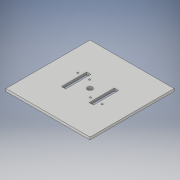
# Autodesk Inventor part: thumper-bumper-base
Saved by Autodesk Inventor 2017 (Build 210142000, 142)
## iProperties
Created: 2017-02-21
Part Number: thumper-bumper-base
Material: Generic
Document SubType Name: Modeling
Designer: John
Density: 1 g/cm^3
Appearance: Default
Author: John
Autodesk Inventor part; units mm, degrees
ref_plane "YZ Plane" through (0, 0, 0) normal (1, 0, 0) x (0, 1, 0)
ref_plane "XZ Plane" through (0, 0, 0) normal (0, 1, 0) x (-1, 0, 0)
ref_plane "XY Plane" through (0, 0, 0) normal (0, 0, 1) x (1, 0, 0)
sketch "Sketch1" plane through (0, 0, 0) normal (0, 1, 0) x (-1, 0, 0)
  line L0 (50, -50) -> (-50, -50)
  line L1 (-50, -50) -> (-50, 50)
  line L2 (-50, 50) -> (50, 50)
  line L3 (50, 50) -> (50, -50)
  line L4 (50, -50) -> (-50, 50) construction
  line L5 (-50, -50) -> (50, 50) construction
  line L6 (-14, -15) -> (-19, -15)
  line L7 (-19, -15) -> (-19, 15)
  line L8 (-19, 15) -> (-14, 15)
  line L9 (-14, 15) -> (-14, -15)
  line L10 (-14, -15) -> (-19, 15) construction
  line L11 (-19, -15) -> (-14, 15) construction
  line L12 (0, -50) -> (0, 50) construction
  line L13 (14, -15) -> (19, -15)
  line L14 (19, -15) -> (19, 15)
  line L15 (19, 15) -> (14, 15)
  line L16 (14, 15) -> (14, -15)
  line L17 (14, -15) -> (19, 15) construction
  line L18 (19, -15) -> (14, 15) construction
  line L19 (-19, 15) -> (-19, 50) construction
  line L20 (-19, -15) -> (-19, -50) construction
  circle A0 centre (0, 0) radius 3
  point P0 (-16.5, 0)
  point P1 (16.5, 0)
  dimension "d0" = 100
  dimension "d1" = 100
  dimension "d4" = 5
  dimension "d5" = 30
  dimension "d6" = 14
  dimension "d21" = 6
  constraints: 42 end point, 8 midpoint, 5 symmetric about line, 4 parallel, 3 perpendicular, 3 point on line, 2 horizontal, 1 centre point, 1 coincident, 1 collinear
  measures "d0" distance of L1.end L2.end
  measures "d1" distance of L0.end L1.end
  measures "d4" distance of L7.end L8.end
  measures "d5" distance of L6.end L7.end
  measures "d6" distance from line of point (0, 0) L9
  measures "d21" diameter of A0
extrude "Extrusion2" add sketch "Sketch1" along normal blind 3
sketch "Sketch2" plane through (0, 3, 0) normal (0, 1, 0) x (1, 0, 0)
  circle A0 centre (23.5, -9) radius 1
  circle A1 centre (9.5, -9) radius 1
  line L0 (23.5, -9) -> (16.5, -9) construction
  line L1 (19, -15) -> (14, -15) construction
  line L2 (16.5, -15) -> (16.5, -9) construction
  line L3 (16.5, -9) -> (9.5, -9) construction
  line L4 (-19, 15) -> (-14, 15) construction
  line L5 (-16.5, 15) -> (-16.5, 9) construction
  line L6 (-16.5, 9) -> (-9.5, 9) construction
  line L7 (-16.5, 9) -> (-23.5, 9) construction
  circle A2 centre (-9.5, 9) radius 1
  circle A3 centre (-23.5, 9) radius 1
  point P0 (0, 0)
  dimension "d11" = 2
  dimension "d12" = 2
  dimension "d13" = 6
  dimension "d14" = 7
  dimension "d17" = 2
  dimension "d18" = 2
  constraints: 12 end point, 4 centre point, 4 equal length, 4 horizontal, 2 coincident, 2 midpoint, 2 vertical
  measures "d11" diameter of A0
  measures "d12" diameter of A1
  measures "d13" distance of L2.start L0.end
  measures "d14" distance of L0.start L0.end
  measures "d17" diameter of A2
  measures "d18" diameter of A3
extrude "Extrusion3" cut sketch "Sketch2" against normal through all
body "Solid2"
